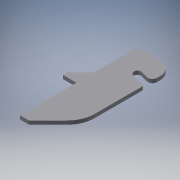
# Autodesk Inventor part: Rear Wheel Holder
Saved by Autodesk Inventor 2018 (Build 220112000, 112)
## iProperties
Created: 2018-08-10
Part Number: Rear Wheel Holder
Material: Generic
Document SubType Name: Modeling
Designer: ruben
Density: 1 g/cm^3
Sheet Metal Rule: Default_mm
Appearance: Default
Author: ruben
Autodesk Inventor part; units mm, degrees
ref_plane "YZ Plane" through (0, 0, 0) normal (1, 0, 0) x (0, 1, 0)
ref_plane "XZ Plane" through (0, 0, 0) normal (0, 1, 0) x (-1, 0, 0)
ref_plane "XY Plane" through (0, 0, 0) normal (0, 0, 1) x (1, 0, 0)
sketch "Sketch3" plane through (0, 0, 0) normal (0, 0, 1) x (1, 0, 0)
  line L0 (-91, 0) -> (91, 0) projected
  line L1 (0, -48.6774) -> (0, 47.0644) projected
  line L2 (65, -10) -> (35, 20)
  line L3 (35, 20) -> (-31.6994, 20)
  line L4 (-31.6994, 20) -> (-36.1448, 3.9333)
  line L5 (65, -20) -> (2.5, -20)
  line L6 (2.5, -20) -> (2.5, -35)
  line L7 (2.5, -35) -> (-2.5, -35)
  line L8 (-2.5, -35) -> (-17.5, -20)
  line L9 (-17.5, -20) -> (-65, -20)
  line L10 (-65, -20) -> (-65, 20)
  line L11 (-65, 20) -> (-40, 20)
  line L12 (65, -20) -> (65, -10)
  line L13 (-40, 20) -> (-43.8552, 6.0667)
  arc A0 (-43.8552, 6.0667) -> (-36.1448, 3.9333) centre (-40, 5) ccw
  line L14 (-26.282, 1.2044) -> (-45.4203, 6.4997) construction
  line L15 (-40, -18.8457) -> (-40, 33.387) construction
  point P0 (0, 0)
  dimension "d0" = 130
  dimension "d1" = 40
  dimension "d2" = 10
  dimension "d4" = 5
  dimension "d5" = 20
  dimension "d6" = 30
  dimension "d8" = 55
  dimension "d11" = 8
  dimension "d12" = 25
  dimension "d16" = 8
  dimension "d23" = 15
  constraints: 28 end point, 4 perpendicular, 4 point on line, 3 parallel, 2 collinear, 2 horizontal, 2 point on circle, 1 centre point, 1 symmetric about line, 1 tangent, 1 vertical, 3 other
  measures "d0" distance between parallel lines of L10 L12
  measures "d1" distance between parallel lines of L3 L9
  measures "d2" distance of L5.start L2.start
  measures "d4" distance of L6.end L7.end
  measures "d5" distance of L8.end L5.end
  measures "d6" horizontal distance of L2.end L2.start
  measures "d8" distance between parallel lines of L11 L7
  measures "d11" distance between parallel lines of L13 L4
  measures "d12" distance from line of L10 L11.end
  measures "d16" distance of L13.end L4.end
  measures "d23" distance from line of L11 A0.centre
extrude "Extrusion1" add sketch "Sketch3" along normal blind 4
fillet "Fillet1" radius 2 2 edges at (-31.6994, 20, 2) (65, -10, 2)
fillet "Fillet2" radius 30 1 edges at (35, 20, 2)
fillet "Fillet3" radius 5 2 edges at (-40, 20, 2) (-65, -20, 2)
fillet "Fillet4" radius 15 1 edges at (-65, 20, 2)
equation "\"BendRadius\" = Thickness"
equation "\"BendReliefWidth\" = Thickness"
equation "\"BendReliefDepth\" = 0.5 * Thickness"
equation "\"CornerReliefSize\" = 4 * Thickness"
equation "\"MinimumRemnant\" = 2 * Thickness"
equation "\"TransitionRadius\" = BendRadius"
equation "\"JacobiRadiusSize\" = BendRadius"
equation "\"GapSize\" = Thickness"
equation "\"Thickness\" = 0.5"
body "Solid1"
